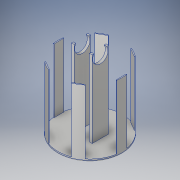
# Autodesk Inventor part: piston holder thing
Saved by Autodesk Inventor 2018 (Build 220112000, 112)
## iProperties
Created: 2018-03-12
Part Number: piston holder thing
Material: Aluminum 6061
Document SubType Name: Modeling
Designer: 238438
Density: 2.7 g/cm^3
Appearance: Aluminum - Flat
Mass: 0.0928884 g
Surface Area: 3.14127 cm^2
Volume: 0.0344031 cm^3
Author: 238438
Autodesk Inventor part; units mm, degrees
ref_plane "YZ Plane" through (0, 0, 0) normal (1, 0, 0) x (0, 1, 0)
ref_plane "XZ Plane" through (0, 0, 0) normal (0, 1, 0) x (-1, 0, 0)
ref_plane "XY Plane" through (0, 0, 0) normal (0, 0, 1) x (1, 0, 0)
sketch "Sketch1" plane through (0, 0, 0) normal (0, 1, 0) x (-1, 0, 0)
  circle A0 centre (0, 0) radius 3.9878
  dimension "d0" = 7.9756
  constraints: 1 centre point, 1 coincident
  measures "d0" diameter of A0
extrude "Extrusion1" add sketch "Sketch1" along normal blind 0.3302
sketch "Sketch2" plane through (0, 0.3302, 0) normal (0, 1, 0) x (1, 0, 0)
  circle A0 centre (0, 0) radius 3.9878 projected
  arc A1 (-3.9382, 0.627) -> (-3.9382, -0.627) centre (0, 0) ccw
  line L0 (-3.9382, -0.627) -> (-3.9382, 0.627) construction
  line L1 (-3.9382, -0.627) -> (-2.6841, -0.627) construction
  line L2 (-3.9382, -0.627) -> (-3.8546, -0.6035)
  line L3 (-3.9382, 0.627) -> (-3.8546, 0.6111)
  line L4 (-3.8546, 0.6111) -> (-3.8546, -0.6035)
  line L5 (-2.4566, -3.0327) -> (-1.4047, -3.64)
  arc A2 (-2.5121, -3.0971) -> (-1.4261, -3.7241) centre (0, 0) ccw
  line L6 (-1.4261, -3.7241) -> (-1.4047, -3.64)
  line L7 (-2.5121, -3.0971) -> (-2.4566, -3.0327)
  line L8 (1.3981, -3.6438) -> (2.45, -3.0365)
  arc A3 (1.4261, -3.7241) -> (2.5121, -3.0971) centre (0, 0) ccw
  line L9 (2.5121, -3.0971) -> (2.45, -3.0365)
  line L10 (1.4261, -3.7241) -> (1.3981, -3.6438)
  line L11 (3.8546, -0.6111) -> (3.8546, 0.6035)
  arc A4 (3.9382, -0.627) -> (3.9382, 0.627) centre (0, 0) ccw
  line L12 (3.9382, 0.627) -> (3.8546, 0.6035)
  line L13 (3.9382, -0.627) -> (3.8546, -0.6111)
  line L14 (2.4566, 3.0327) -> (1.4047, 3.64)
  arc A5 (2.5121, 3.0971) -> (1.4261, 3.7241) centre (0, 0) ccw
  line L15 (1.4261, 3.7241) -> (1.4047, 3.64)
  line L16 (2.5121, 3.0971) -> (2.4566, 3.0327)
  line L17 (-1.3981, 3.6438) -> (-2.45, 3.0365)
  arc A6 (-1.4261, 3.7241) -> (-2.5121, 3.0971) centre (0, 0) ccw
  line L18 (-2.5121, 3.0971) -> (-2.45, 3.0365)
  line L19 (-1.4261, 3.7241) -> (-1.3981, 3.6438)
  dimension "d3" = 90
  dimension "d6" = 360
  constraints: 40 end point, 14 point on circle, 6 centre point, 2 perpendicular, 1 horizontal, 55 other
  measures "d3" angle of L1 L0
extrude "Extrusion2" add sketch "Sketch2" along normal blind 7.9248 contours A0 L13 L11 L12 | L16 L14 L15 A0 | A0 L10 L8 L9 | L19 L17 L18 A0 | A0 L7 L5 L6 | L3 L4 L2 A0
fillet "Fillet1" radius 0.1905 1 edges at (3.9878, 0, 0)
sketch "Sketch3" plane through (0, 0.3302, 0) normal (0, 1, 0) x (1, 0, 0)
  line L0 (-0.9525, 1.016) -> (-1.2827, 1.016)
  line L1 (-1.2827, 1.016) -> (-1.2827, -1.016)
  line L2 (-1.2827, -1.016) -> (-0.9525, -1.016)
  line L3 (-0.9525, -1.016) -> (-0.9525, 1.016)
  line L4 (0, 2.5556) -> (0, -1.5997)
  line L5 (0.9525, 1.016) -> (1.2827, 1.016)
  line L6 (1.2827, 1.016) -> (1.2827, -1.016)
  line L7 (1.2827, -1.016) -> (0.9525, -1.016)
  line L8 (0.9525, -1.016) -> (0.9525, 1.016)
  point P0 (0, 0)
  dimension "d11" = 0.3302
  dimension "d12" = 2.032
  dimension "d13" = 1.016
  dimension "d14" = 0.9525
  constraints: 18 end point, 4 symmetric about line, 2 parallel, 1 horizontal, 1 perpendicular, 1 vertical
  measures "d11" distance of L2.end L1.end
  measures "d12" distance between parallel lines of L2 L0
  measures "d13" vertical distance of point (0, 0) L0.start
  measures "d14" distance from line of L3 point (0, 0)
extrude "Extrusion3" add sketch "Sketch3" along normal blind 9.525
sketch "Sketch5" plane through (1.2827, 0.3302, 1.016) normal (1, 0, 0) x (0, 0, -1)
  circle A0 centre (1.016, 9.0059) radius 0.9525
  point P0 (1.016, -0.3302)
  dimension "d18" = 1.905
  constraints: 1 centre point
  measures "d18" diameter of A0
extrude "Extrusion4" cut sketch "Sketch5" against normal through all
body "Solid1"
